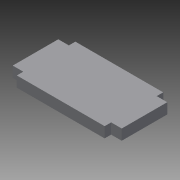
# Autodesk Inventor part: arm-servo
Saved by Autodesk Inventor 2013 (Build 170138000, 138)
## iProperties
Created: 2012-09-08
Part Number: arm-servo
Material: Generic
Document SubType Name: Modeling
Designer: frankenteddy
Density: 1 g/cm^3
Author: frankenteddy
Autodesk Inventor part; units mm, degrees
ref_plane "YZ Plane" through (0, 0, 0) normal (1, 0, 0) x (0, 1, 0)
ref_plane "XZ Plane" through (0, 0, 0) normal (0, 1, 0) x (-1, 0, 0)
ref_plane "XY Plane" through (0, 0, 0) normal (0, 0, 1) x (1, 0, 0)
sketch "Block1" plane through (0, 0, 0) normal (0, 0, 1) x (1, 0, 0)
  circle A0 centre (74.029, 24.2723) radius 1
  line L0 (49.279, 30.4723) -> (71.779, 30.4723)
  line L1 (71.779, 30.4723) -> (71.779, 18.0723)
  line L2 (71.779, 18.0723) -> (49.279, 18.0723)
  line L3 (49.279, 18.0723) -> (49.279, 30.4723)
  line L4 (49.279, 30.4723) -> (44.779, 30.4723)
  line L5 (44.779, 30.4723) -> (44.779, 18.0723)
  line L6 (44.779, 18.0723) -> (49.279, 18.0723)
  line L7 (49.279, 18.0723) -> (49.279, 30.4723)
  line L8 (71.779, 30.4723) -> (76.279, 30.4723)
  line L9 (76.279, 30.4723) -> (76.279, 18.0723)
  line L10 (76.279, 18.0723) -> (71.779, 18.0723)
  line L11 (71.779, 18.0723) -> (71.779, 30.4723)
  line L12 (44.779, 24.2723) -> (76.279, 24.2723) construction
  line L13 (47.029, 30.4723) -> (47.029, 18.0723) construction
  circle A1 centre (47.029, 24.2723) radius 1
  line L14 (74.029, 30.4723) -> (74.029, 18.0723) construction
  point P0 (60.979, 24.0984)
  dimension "d7" = 22.5
  dimension "d8" = 12.4
  dimension "d9" = 4.5
  dimension "d10" = 4.5
  dimension "d11" = 2
  dimension "d12" = 2
  measures "d7" distance of L1.end L2.end
  measures "d8" distance of L0.end L1.end
  measures "d9" distance of L6.end L5.end
  measures "d10" distance of L9.end L10.end
  measures "d11" diameter of A0
  measures "d12" diameter of A1
sketch "Sketch1" plane through (0, 0, 0) normal (0, 0, 1) x (1, 0, 0)
  line L0 (-92.7646, -8.503) -> (-89.7646, -8.503)
  line L1 (-89.7646, -8.503) -> (-89.7646, -11.753)
  line L2 (-89.7646, -11.753) -> (-92.7646, -11.753)
  line L3 (-92.7646, -11.753) -> (-92.7646, -8.503)
  line L4 (-92.7646, -21.6527) -> (-89.7646, -21.6527)
  line L5 (-89.7646, -21.6527) -> (-89.7646, -21.7527)
  line L6 (-89.7646, -21.7527) -> (-92.7646, -21.7527)
  line L7 (-92.7646, -21.7527) -> (-92.7646, -21.6527)
  line L8 (-26.7369, 26.8899) -> (0.2631, 26.8899)
  line L9 (0.2631, 26.8899) -> (0.2631, 8.8899)
  line L10 (0.2631, 8.8899) -> (-26.7369, 8.8899)
  line L11 (-26.7369, 8.8899) -> (-26.7369, 26.8899)
  line L12 (-29.9869, 24.8899) -> (-26.7369, 24.8899)
  line L13 (-26.7369, 24.8899) -> (-26.7369, 10.8899)
  line L14 (-26.7369, 10.8899) -> (-29.9869, 10.8899)
  line L15 (-29.9869, 10.8899) -> (-29.9869, 24.8899)
  line L16 (-29.9869, 17.8899) -> (-26.7369, 17.8899) construction
  line L17 (-26.7369, 17.8899) -> (0.2631, 17.8899) construction
  line L18 (-13.2369, 26.8899) -> (-13.2369, 8.8899) construction
  line L19 (3.5131, 24.8899) -> (0.2631, 24.8899)
  line L20 (0.2631, 24.8899) -> (0.2631, 10.8899)
  line L21 (0.2631, 10.8899) -> (3.5131, 10.8899)
  line L22 (3.5131, 10.8899) -> (3.5131, 24.8899)
  line L23 (3.5131, 17.8899) -> (0.2631, 17.8899) construction
  point P0 (0, 0)
  dimension "d0" = 3
  dimension "mat" = 3.25
  dimension "d2" = 3
  dimension "d3" = 0.1
  dimension "d42" = 27
  dimension "d43" = 18
  dimension "d44" = 3.25
  dimension "d45" = 14
  constraints: 48 end point, 8 parallel, 7 symmetric about line, 6 midpoint, 4 horizontal, 4 perpendicular, 2 collinear
  measures "d0" distance of L1.end L3.start
  measures "mat" distance of L1.start L1.end
  measures "d2" distance of L5.end L7.start
  measures "d3" distance of L5.start L5.end
  measures "d42" distance of L9.end L10.end
  measures "d43" distance of L8.end L9.end
  measures "d44" distance of L13.end L14.end
  measures "d45" distance of L12.end L13.end
extrude "Extrusion6" add sketch "Sketch1" along normal blind 3.25 contours L8 L9 L10 L11 | L11 L14 L15 L12 | L19 L22 L21 L9
equation "\"d44\" = mat"
equation "\"d46\" = mat"
body "Solid6"
